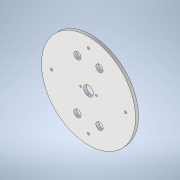
# Autodesk Inventor part: Base3
Saved by Autodesk Inventor 2022 (Build 260153000, 153)
## iProperties
Created: 2021-09-09
Part Number: Base3
Material: Generic
Document SubType Name: Modeling
Designer: Administrador
Density: 1 g/cm^3
Appearance: Default
Author: Administrador
Autodesk Inventor part; units mm, degrees
ref_plane "YZ Plane" through (0, 0, 0) normal (1, 0, 0) x (0, 1, 0)
ref_plane "XZ Plane" through (0, 0, 0) normal (0, 1, 0) x (-1, 0, 0)
ref_plane "XY Plane" through (0, 0, 0) normal (0, 0, 1) x (1, 0, 0)
sketch "Sketch1" plane through (0, 0, 0) normal (0, 0, 1) x (1, 0, 0)
  circle A0 centre (0, 0) radius 47
  circle A1 centre (0, 0) radius 4.95
  circle A2 centre (0, 0) radius 37 construction
  circle A3 centre (0, 37) radius 1.25
  circle A4 centre (37, 0) radius 1.25
  circle A5 centre (0, -37) radius 1.25
  circle A6 centre (-37, 0) radius 1.25
  line L0 (0, 0) -> (0, 25) construction
  line L1 (0, 25) -> (11, 25) construction
  circle A7 centre (11, 25) radius 3.625
  line L2 (11, 25) -> (-11, 25) construction
  line L3 (-11, 25) -> (-11, -25) construction
  line L4 (-11, -25) -> (11, -25) construction
  line L5 (11, -25) -> (11, 25) construction
  circle A8 centre (-11, 25) radius 3.625
  circle A9 centre (-11, -25) radius 3.625
  circle A10 centre (11, -25) radius 3.625
  line L6 (0, 0) -> (-7.9, 0) construction
  line L7 (-7.9, 0) -> (7.9, 0) construction
  circle A11 centre (-7.9, 0) radius 0.975
  circle A12 centre (7.9, 0) radius 0.975
  point P0 (47, 0)
  dimension "d0" = 94
  dimension "d1" = 9.9
  dimension "d4" = 74
  dimension "d5" = 2.5
  dimension "d6" = 2.5
  dimension "d7" = 2.5
  dimension "d8" = 2.5
  dimension "d9" = 25
  dimension "d10" = 11
  dimension "d11" = 7.25
  dimension "d12" = 22
  dimension "d13" = 50
  dimension "d14" = 7.9
  dimension "d15" = 15.8
  dimension "d16" = 1.95
  dimension "d17" = 1.95
  constraints: 16 end point, 12 centre point, 10 coincident, 4 point on circle, 3 horizontal, 2 parallel, 1 horizontal alignment, 1 perpendicular, 1 point on line, 1 vertical, 2 other
  measures "d1" diameter of A1
  measures "d4" diameter of A2
  measures "d5" diameter of A3
  measures "d6" diameter of A4
  measures "d7" diameter of A5
  measures "d8" diameter of A6
  measures "d9" distance of L0.start L0.end
  measures "d10" distance of L0.end L1.end
  measures "d11" diameter of A7
  measures "d12" distance of L4.end L3.end
  measures "d13" distance of L3.end L2.end
  measures "d14" distance of L0.start L6.end
  measures "d15" distance of L6.end L7.end
  measures "d16" diameter of A11
  measures "d17" diameter of A12
extrude "Extrusion1" add sketch "Sketch1" along normal blind 3
body "Solid1"
